LinksPassive 4 to print_v1 (Autodesk Fusion 360 design; units mm, degrees)
Autodesk Fusion 360 part; units mm, degrees
sketch "most" plane through (0, 0, 0) normal (0, 0, 1) x (1, 0, 0)
  line L0 (-18.5, 6) -> (-18.5, -6) construction
  line L1 (18.5, -6) -> (18.5, 6) construction
  line L2 (18.5, 6) -> (-18.5, -6) construction
  line L3 (-18.5, 6) -> (18.5, -6) construction
  circle A0 centre (12.5, 0) radius 0.975
  circle A1 centre (12.5, 0) radius 2.975
  circle A2 centre (12.5, 0) radius 6
  line L4 (0, 6) -> (0, -15) construction
  line L5 (12.5, 6) -> (0, 6)
  line L6 (0, -6) -> (12.5, -6)
  line L7 (12.5, -6) -> (12.5, 6)
  line L8 (12.5, 6) -> (-12.5, -6) construction
  line L9 (-12.5, 6) -> (12.5, -6) construction
  line L10 (18.5, 6) -> (0, 6) construction
  line L11 (-12.5, 6) -> (-18.5, 6) construction
  line L12 (-18.5, -6) -> (-12.5, -6) construction
  line L13 (0, -6) -> (18.5, -6) construction
  line L14 (0, -6) -> (-18.5, -6) construction
  line L15 (-12.5, -6) -> (-12.5, 6)
  line L16 (-18.5, 6) -> (0, 6) construction
  circle A3 centre (-12.5, 0) radius 6
  circle A4 centre (-12.5, 0) radius 2.975
  circle A5 centre (-12.5, 0) radius 0.975
  line L17 (0, -6) -> (-12.5, -6)
  line L18 (-12.5, 6) -> (0, 6)
  dimension "d2" = 12
  dimension "d3" = 1.95
  dimension "d4" = 5.95
  dimension "d5" = 12
  dimension "d6" = 12.5
  dimension "d7" = 25
  dimension "d45" = 7
  constraint horizontal L10
  constraint perpendicular L0 L10
  constraint parallel L10 L12
  constraint parallel L0 L1
  constraint coincident L2 origin
  constraint coincident L3 origin
  constraint concentric A0 A1
  constraint concentric A0 A2
  constraint perpendicular L4 L12
  constraint horizontal origin A0.centre
  constraint horizontal L5
  constraint parallel L5 L6
  constraint coincident A2 L5.start
  constraint coincident L8 origin
  constraint coincident L9 origin
  constraint collinear L10 L11
  constraint coincident L4 L6.start
  constraint collinear L12 L13
  constraint symmetric L1.end L4 L0.start
  constraint symmetric L1.start L4 L0.end
  constraint symmetric A0 L4 A5
  constraint symmetric A1 L4 A4
  constraint symmetric A2 L4 A3
  constraint symmetric L4 L5.start L9.start
  constraint symmetric L4 L6.end L8.end
  constraint symmetric L4 L5.end L10.end
  constraint symmetric L4 L6.start L13.start
  constraint perpendicular L15 L18
  measures "d2" distance of L0.start L0.end
  measures "d3" diameter of A0
  measures "d4" diameter of A1
  measures "d5" diameter of A2
  measures "d6" distance of origin A0.centre
  measures "d7" distance of L8.end L6.end
extrude "base" add sketch "most" along normal mid plane 10 contours A0 L7 | A0 A1 L7 | A1 A2 L7 | A2 L5 L6 A3 L17 L18 | L15 A3 A4 | L15 A4 A5 | L15 A5 picked at (11.8524, -0.1625) picked at (11.328, -1.9813) picked at (9.947, 4.2738) picked at (-7.5388, -0.4258) picked at (-10.2051, -0.1874) picked at (-11.9343, -0.135)
extrude "r big cyl" add sketch "most" along normal blind 7 and the other way blind 5 contours A0 A1 L7 | A0 A1 L7 | A1 A2 L7 | A1 A2 L7
extrude "r small cyl" add sketch "most" along normal blind 12 and the other way blind 5 contours A0 A1 L7 | A0 A1 L7
extrude "l  big cyl" add sketch "most" along normal blind -7 and the other way blind -5 contours L15 A3 A4 | L15 A3 A4 | L15 A4 A5 | L15 A4 A5
extrude "Extrude7" add sketch "most" against normal blind 12 contours L15 A4 A5 | L15 A4 A5
extrude "Extrude8" cut sketch "most" along normal blind 5 and the other way blind 12 contours L15 A5 | L15 A5
extrude "Extrude9" cut sketch "most" along normal blind 12 and the other way blind 5 contours A0 L7 | A0 L7
fillet "Fillet1" radius 0.3 1 edges at (9.7263, -1.0758, 12)
sketch "top nut" plane through (0, 0, 5) normal (0, 0, 1) x (-1, 0, 0)
  line L0 (12.5, 6) -> (-12.5, 6)
  arc A0 (-12.5, -6) -> (-12.5, 6) centre (-12.5, 0) ccw
  line L1 (-12.5, -6) -> (12.5, -6)
  circle A1 centre (12.5, 0) radius 2.5 construction
  line L2 (14.5842, -1.3806) -> (14.7377, 1.1147)
  line L3 (14.7377, 1.1147) -> (12.6535, 2.4953)
  line L4 (12.6535, 2.4953) -> (10.4158, 1.3806)
  line L5 (10.4158, 1.3806) -> (10.2623, -1.1147)
  line L6 (10.2623, -1.1147) -> (12.3465, -2.4953)
  line L7 (12.3465, -2.4953) -> (14.5842, -1.3806)
  circle A2 centre (12.5, 0) radius 0.975
  arc A3 (12.5, -6) -> (12.5, 6) centre (12.5, 0) ccw
  point P0 (12.5, 0)
  dimension "d35" = 5
  constraint coincident P0 A1.centre
  constraint coincident A1 L2.start
  measures "d35" diameter of A1
extrude "Extrude10" cut sketch "top nut" against normal blind 4 contours L2 L3 L4 L5 L6 L7
sketch "bottom nut" plane through (0, 0, -5) normal (0, 0, -1) x (1, 0, 0)
  circle A0 centre (12.5, 0) radius 2.5 construction
  arc A1 (-12.5, -6) -> (-12.5, 6) centre (-12.5, 0) ccw
  line L0 (-12.5, -6) -> (12.5, -6)
  line L1 (12.5, 6) -> (-12.5, 6)
  circle A2 centre (12.5, 0) radius 0.975
  arc A3 (12.5, -6) -> (12.5, 6) centre (12.5, 0) ccw
  line L2 (12.5, -2.5) -> (14.6651, -1.25)
  line L3 (14.6651, -1.25) -> (14.6651, 1.25)
  line L4 (14.6651, 1.25) -> (12.5, 2.5)
  line L5 (12.5, 2.5) -> (10.3349, 1.25)
  line L6 (10.3349, 1.25) -> (10.3349, -1.25)
  line L7 (10.3349, -1.25) -> (12.5, -2.5)
  point P0 (12.5, 0)
  point P1 (12.5, 0)
  dimension "d38" = 5
  constraint coincident P0 A0.centre
  constraint coincident P1 P0
  constraint coincident A0 L2.start
  measures "d38" diameter of A0
extrude "Extrude11" cut sketch "bottom nut" against normal blind 4 contours A2 | L2 L3 L4 L5 L6 L7
fillet "Fillet4" radius 0.3 1 edges at (-15.2737, 1.0758, -12)
equation "d2 = BigBarrelDiam"
equation "d3 = smallerHoleDiam"
equation "d4 = nipDiameter"
equation "d5 = BigBarrelDiam"
equation "d8 = rect / 2"
equation "d10 = rect / 2 + shoulder"
equation "d12 = rect + shoulder"
equation "d16 = -rect / 2 - shoulder"
equation "d20 = -rect - shoulder"
equation "d22 = rect / 2"
equation "d24 = rect + shoulder"
equation "d25 = 0.0 °"
equation "d26 = rect + shoulder"
equation "d36 = -hex"
equation "d39 = -hex"
equation "d48 = rect / 2"
equation "d49 = 0.0 °"
equation "d50 = rect / 2"
equation "d51 = 0.0 °"
equation "d52 = -rect / 2"
equation "d53 = 0.0 °"
equation "d54 = rect / 2"
equation "d55 = 0.0 °"
equation "rect = 10 mm"
equation "shoulder = 2 mm"
equation "nip = 4 mm"
equation "hex = 4 mm"
equation "nipDiameter = 5.95 mm"
equation "BigBarrelDiam = 12 mm"
equation "smallerHoleDiam = 1.95 mm"
